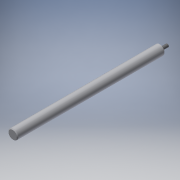
# Autodesk Inventor part: 22-130 RAIL
Saved by Autodesk Inventor 2018 (Build 220105000, 105)
## iProperties
Created: 2004-11-24
Part Number: 22-130 RAIL
Material: Aluminum-6061
Document SubType Name: Modeling
Designer: Autodesk, Inc.
Manufacturer: Standard
Standards Organization: Custom
Description: BIN MOUNTING SLIDE RAIL
Catalog Web Link: http://www.parker.com/ead/cm1.asp?cmid=809
Vendor: PARKER IPS
Mass: 524.122 g
Surface Area: 317.4 cm^2
Volume: 193.403 cm^3
Density: 2.71 g/cm^3
Appearance: Aluminum - Flat
CAGE: 1LJX3
Dept. ID: Product Design
Description #2: ---
Finish #1: ---
Finish #2: ---
Material ID: ---
Project Number: ---
Author: Autodesk, Inc.
Autodesk Inventor part; units mm, degrees
ref_plane "YZ Plane" through (0, 0, 0) normal (1, 0, 0) x (0, 1, 0)
ref_plane "XZ Plane" through (0, 0, 0) normal (0, 1, 0) x (-1, 0, 0)
ref_plane "XY Plane" through (0, 0, 0) normal (0, 0, 1) x (1, 0, 0)
sketch "Sketch1" plane through (0, 0, 0) normal (0, 0, 1) x (1, 0, 0)
  circle A0 centre (0, 0) radius 12.7
  dimension "d0" = 25.4
  constraints: 1 centre point, 1 other
  measures "d0" diameter of A0
extrude "Extrusion1" add sketch "Sketch1" along normal blind 380
sketch "Sketch2" plane through (0, 0, 0) normal (0, 0, -1) x (-1, 0, 0)
  circle A0 centre (0, 0) radius 12.7 construction
  circle A1 centre (0, 0) radius 4
  dimension "d3" = 8
  constraints: 1 centre point, 1 coincident
  measures "d3" diameter of A1
extrude "Extrusion2" add sketch "Sketch2" along normal blind 20
thread "Thread1" size "M8x1.25" class "6g" standard "ANSI Metric M Profile" full length
chamfer "Chamfer1" distance 2 angle 45 1 edges at (-12.7, 0, 380)
body "Solid1"
